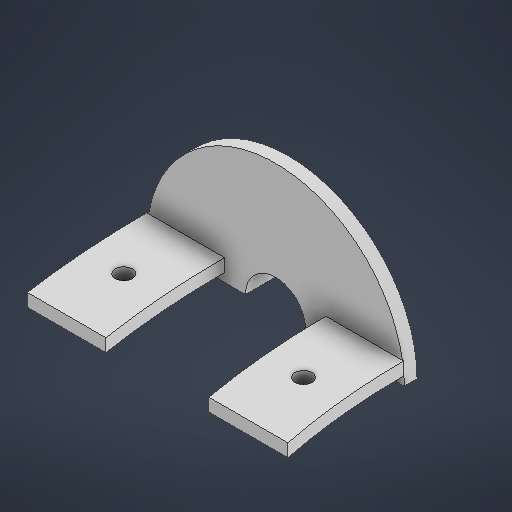
# Autodesk Inventor part: Verbindungsstück-rechts-15mm-Ph-L
Saved by Autodesk Inventor 2026.1 (Build 301233000, 233)
## iProperties
Created: 2025-11-03
Part Number: Verbindungsstück-rechts-15mm-Ph-L
Material: Generisch
Document SubType Name: Modeling
Designer: rebsa
Density: 1 g/cm^3
Appearance: Vorgabe
Author: rebsa
Autodesk Inventor part; units mm, degrees
ref_plane "YZ Plane" through (0, 0, 0) normal (1, 0, 0) x (0, 1, 0)
ref_plane "XZ Plane" through (0, 0, 0) normal (0, 1, 0) x (-1, 0, 0)
ref_plane "XY Plane" through (0, 0, 0) normal (0, 0, 1) x (1, 0, 0)
sketch "Skizze1" plane through (0, 0, 0) normal (0, 1, 0) x (-1, 0, 0)
  circle A0 centre (0, 0) radius 30
  circle A1 centre (0, 0) radius 7
  line L0 (7, 0) -> (30, 0)
  line L1 (-7, 0) -> (-30, 0)
  line L2 (42, 0) -> (-42, 0) projected
  line L3 (0, -42) -> (0, 42) projected
  dimension "d0" = 60
  dimension "d1" = 14
  dimension "d2" = 0
  constraints: 4 end point, 4 point on circle, 2 centre point, 2 point on line, 1 coincident, 1 concentric, 1 horizontal
  measures "d0" diameter of A0
  measures "d1" diameter of A1
  measures "d2" distance between parallel lines of L2 L1
extrude "Extrusion1" add sketch "Skizze1" along normal blind 3 contours L0 A1 L3 A0 | L3 A1 L1 A0 picked at (15.508, 15.8775) picked at (-21.0338, 7.0833)
sketch "Skizze3" plane through (0, 3, 0) normal (0, 1, 0) x (1, 0, 0)
  circle A0 centre (0, 0) radius 7.9
  circle A1 centre (0, 0) radius 7
  arc A2 (-7, 0) -> (7, 0) centre (0, 0) ccw projected
  line L0 (30, 0) -> (7, 0) projected
  line L1 (7.9, 0) -> (-7.9, 0)
  dimension "d13" = 15.8
  constraints: 2 centre point, 2 concentric, 2 end point, 2 point on circle, 1 coincident, 1 collinear, 1 point on line
  measures "d13" diameter of A0
extrude "Extrusion3" add sketch "Skizze3" along normal blind 15 contours A0 L1 A1 L0 picked at (7.5235, -0.6302)
sketch "Skizze4" plane through (-7, 0, 0) normal (0, 0, -1) x (-1, 0, 0)
  circle A0 centre (-186.9335, 0) radius 209.9335
  line L0 (106.9734, 0) -> (-480.8404, 0) projected
  line L1 (-7, -293.9069) -> (-7, 293.9069) projected
  line L2 (23, 0) -> (23, 3) projected
  circle A1 centre (-186.9335, 0) radius 191.832
  circle A2 centre (-186.9335, 0) radius 168.168
  circle A3 centre (-186.9335, 0) radius 150.0665
  line L3 (-39.8962, -30) -> (20.8454, -30)
  line L4 (2.5382, -30) -> (20.8454, -30)
  line L5 (-21.463, -30) -> (-39.8962, -30)
  point P0 (-7, 0)
  point P1 (4.8985, 0)
  point P2 (-18.7655, 0)
  point P3 (-36.867, 0)
  dimension "d16" = 419.867
  dimension "d17" = 383.664
  dimension "d18" = 336.336
  dimension "d19" = 300.133
  dimension "d20" = 30
  constraints: 6 end point, 2 collinear, 2 point on line, 1 midpoint, 1 perpendicular, 1 vertical, 12 other
  measures "d20" distance between parallel lines of L3 L0
extrude "Extrusion4" add sketch "Skizze4" against normal blind 5 contours L3 A1 L0 A0 | L3 A3 L0 A2 picked at (-33.1917, -26.6918)
sketch "Skizze5" plane through (-7.9, 3, 0) normal (0, 0, -1) x (-1, 0, 0)
  circle A0 centre (-187.8335, -3) radius 209.9335
  line L0 (22.1, -3) -> (22.1, 0)
  circle A1 centre (-187.8335, -3) radius 191.832
  circle A2 centre (-187.8335, -3) radius 168.168
  circle A3 centre (-187.8335, -3) radius 150.0665
  arc A4 (19.9454, -33) -> (22.1, -3) centre (-187.8335, -3) ccw projected
  line L1 (1.6382, -33) -> (19.9454, -33) projected
  line L2 (19.9454, -33) -> (1.6382, -33)
  line L3 (1.6382, -33) -> (-22.363, -33)
  line L4 (-40.7962, -33) -> (-22.363, -33)
  line L5 (22.1, -3) -> (3.9985, -3)
  line L6 (21.6804, -3) -> (-37.4804, -3) projected
  line L7 (-19.6655, -3) -> (-37.767, -3)
  point P0 (-7.9, -3)
  point P1 (193.7355, 3.1959)
  point P2 (175.634, 3.1959)
  point P3 (151.97, 3.1959)
  point P4 (133.8685, 3.1959)
  point P5 (19.9454, -33)
  dimension "d23" = 419.867
  dimension "d24" = 383.664
  dimension "d25" = 336.336
  dimension "d26" = 300.133
  constraints: 12 end point, 5 point on circle, 5 point on line, 4 centre point, 3 concentric, 2 collinear, 2 tangent
  measures "d23" diameter of A0
  measures "d24" diameter of A1
  measures "d25" diameter of A2
  measures "d26" diameter of A3
extrude "Extrusion5" cut sketch "Skizze5" against normal blind 2 contours A0 L1 A1 L5 | L4 A3 L7 L6 A2 picked at (8.1773, -29.6819) picked at (-34.0917, -29.6918)
sketch "Skizze6" plane through (-7, 0, 5) normal (0, 0, 1) x (1, 0, 0)
  line L0 (36.5804, 0) -> (-22.5804, 0) projected
  line L1 (-23, 0) -> (-23, 3) projected
  circle A0 centre (186.9335, 0) radius 200.8827
  arc A1 (-23, 0) -> (-20.8454, -30) centre (186.9335, 0) ccw projected
  circle A2 centre (186.9335, 0) radius 159.1173
  point P0 (7, 0)
  point P1 (-13.3884, -15)
  point P2 (28.5249, -15)
  dimension "d32" = 401.7655
  dimension "d33" = 318.2345
  dimension "d30" = 15
  dimension "d34" = 15
  constraints: 7 other
  measures "d30" distance from line of L0 point (-13.388, -15)
  measures "d34" distance from line of L0 point (28.525, -15)
hole "Bohrung1" at (-20.3884, -15, 5) at (21.5249, -15, 5) direction (0, 0, -1) diameter 4 depth 10 tip angle 118
